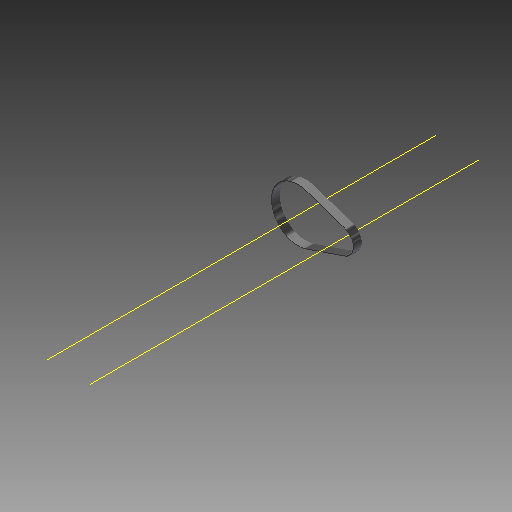
# Autodesk Inventor part: Zahnriemen
Saved by Autodesk Inventor 2018.3 (Build 223284000, 284)
## iProperties
Created: 2018-08-12
Part Number: Zahnriemen
Material: Rubber
Document SubType Name: Modeling
Designer: JochenAlt
Density: 1 g/cm^3
Appearance: Rubber - Black - Version 1.1
CustomPartVersion: 1
Author: JochenAlt
Autodesk Inventor part; units mm, degrees
sketch "Skizzenpfad" plane through (0, 0, 0) normal (0, 0, 1) x (1, 0, 0)
  arc A0 (-93.5818, 18.8306) -> (-93.5818, -18.8306) centre (-100, 0) ccw
  arc A1 (-64.8529, -9.0387) -> (-64.8529, 9.0387) centre (-67.9337, 0) ccw
  line L0 (-64.8529, -9.0387) -> (-93.5818, -18.8306)
  line L1 (-93.5818, 18.8306) -> (-64.8529, 9.0387)
  constraints: 4 end point, 4 point on circle, 2 centre point
ref_plane "Querschnittsebene" through (-93.5818, -18.8306, 0) normal (0.9465, 0.3226, 0) x (0, 0, 1)
ref_plane "Arbeitsebene2" through (-100, 0, 0) normal (-1, 0, 0) x (0, 0, 1)
ref_plane "Arbeitsebene3" through (-67.9337, 0, 0) normal (-0.9239, 0.3827, 0) x (0, 0, 1)
sketch "Querschnitt" plane through (-93.5818, -18.8306, 0) normal (0.9465, 0.3226, 0) x (0, 0, 1)
  line L0 (-3, 0.3) -> (3, 0.3)
  line L1 (3, 0.3) -> (3, -0.3)
  line L2 (3, -0.3) -> (-3, -0.3)
  line L3 (-3, -0.3) -> (-3, 0.3)
  line L4 (-3, 0) -> (3, 0) construction
  point P0 (0, 0)
  point P1 (0, 0)
  dimension "d0" = 6
  dimension "d4" = 0.3
  dimension "d5" = 0.3
  constraints: 10 end point, 3 midpoint, 2 parallel, 1 coincident, 1 horizontal, 1 perpendicular, 1 other
  measures "d0" distance between parallel lines of L1 L3
  measures "d4" distance between parallel lines of L2 L4
  measures "d5" distance between parallel lines of L4 L0
sweep "Riemen" add profiles "Querschnitt" path "Skizzenpfad"
equation "\"d0\" = da_B"
equation "\"d4\" = da_a"
equation "\"d5\" = da_a2"
equation "\"da_B\" = 6"
equation "\"da_pb\" = 2.5"
equation "\"da_a\" = 0.3"
equation "\"da_S\" = 1.5"
equation "\"da_Beta\" = 20deg"
equation "\"da_Ht\" = 0.7"
equation "\"da_H\" = 1.3"
equation "\"da_a2\" = 0.3"
body "Solid1"
